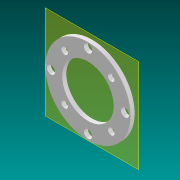
# Autodesk Inventor part: gearboxspacer
Saved by Autodesk Inventor 2020.3 (Build 243373000, 373)
## iProperties
Created: 2020-05-24
Part Number: gearboxspacer
Material: Generic
Document SubType Name: Modeling
Designer: Svend
Density: 1 g/cm^3
Appearance: Default
Author: Svend
Autodesk Inventor part; units mm, degrees
ref_plane "YZ Plane" through (0, 0, 0) normal (1, 0, 0) x (0, 1, 0)
ref_plane "XZ Plane" through (0, 0, 0) normal (0, 1, 0) x (-1, 0, 0)
ref_plane "XY Plane" through (0, 0, 0) normal (0, 0, 1) x (1, 0, 0)
ref_plane "Work Plane1" through (0, 0, 0) normal (0, 0, 1) x (1, 0, 0)
sketch "Sketch1" plane through (0, 0, 0) normal (0, 0, 1) x (1, 0, 0)
  circle A0 centre (0, 0) radius 12.5 projected
  circle A1 centre (0, -18) radius 2 projected
  circle A2 centre (0, 18) radius 2 projected
  circle A3 centre (-18, 0) radius 2 projected
  circle A4 centre (18, 0) radius 2 projected
  circle A5 centre (11.3137, 11.3137) radius 1.6 projected
  circle A6 centre (-11.3137, -11.3137) radius 1.6 projected
  circle A7 centre (-11.3137, 11.3137) radius 1.6 projected
  circle A8 centre (11.3137, -11.3137) radius 1.6 projected
  circle A9 centre (0, 0) radius 20.7 projected
ref_plane "Work Plane2" through (-10.1976, -10.1976, 2) normal (0, 0, 1) x (0.910504, -0.4135003, 0)
extrude "Extrusion1" add sketch "Sketch1" along normal up to surface (2 mm away)
chamfer "Chamfer1" distance 0.2 angle 45 20 edges at (-20.7, 0, 0) (-20.7, 0, 2) (9.7137, -11.3137, 0) (9.7137, -11.3137, 2) (-12.9137, 11.3137, 0) (-12.9137, 11.3137, 2) (-12.9137, -11.3137, 0) (-12.9137, -11.3137, 2) (9.7137, 11.3137, 0) (9.7137, 11.3137, 2) (16, 0, 0) (16, 0, 2) (-20, 0, 0) (-20, 0, 2) (-2, 18, 0) (-2, 18, 2) (-2, -18, 0) (-2, -18, 2) (-12.5, 0, 0) (-12.5, 0, 2)
body "Solid1"
